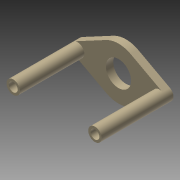
# Autodesk Inventor part: Encoder Mount
Saved by Autodesk Inventor 2013 (Build 170138000, 138)
## iProperties
Created: 2013-06-25
Part Number: Encoder Mount
Material: Generic
Document SubType Name: Modeling
Designer: mvarma
Density: 1 g/cm^3
Author: mvarma
Autodesk Inventor part; units mm, degrees
ref_plane "YZ Plane" through (0, 0, 0) normal (1, 0, 0) x (0, 1, 0)
ref_plane "XZ Plane" through (0, 0, 0) normal (0, 1, 0) x (-1, 0, 0)
ref_plane "XY Plane" through (0, 0, 0) normal (0, 0, 1) x (1, 0, 0)
sketch "Sketch1" plane through (0, 0, 0) normal (0, 0, 1) x (1, 0, 0)
  arc A0 (0, 5.3975) -> (0, -5.3975) centre (0, 0) ccw
  arc A1 (0, 11.1125) -> (0, -11.1125) centre (0, 0) ccw
  circle A2 centre (-17.4625, 0) radius 2.8702
  circle A3 centre (0, 0) radius 17.4625 construction
  line L0 (-17.4625, 0) -> (0, 0) construction
  line L1 (-18.8172, 2.5304) -> (-5.2451, 9.7968)
  line L2 (0, 0) -> (0, 11.1125)
  line L3 (0, 0) -> (0, -11.1125)
  line L4 (-18.8172, -2.5304) -> (-5.2451, -9.7968)
  dimension "d2" = 34.925
  dimension "d0" = 10.795
  dimension "d1" = 22.225
  dimension "d3" = 5.7404
  constraints: 10 end point, 8 point on circle, 4 coincident, 4 tangent, 3 centre point, 2 point on line, 1 collinear, 1 horizontal, 1 horizontal alignment, 1 perpendicular, 2 other
  measures "d0" diameter of A0
  measures "d1" diameter of A1
  measures "d3" diameter of A2
extrude "Extrusion1" add sketch "Sketch1" along normal blind 3.175 contours A0 L3 A1 L2 | A1 L4 A2 L1 | A2
extrude "Extrusion2" add sketch "Sketch1" along normal blind 30.7023 contours A2
hole "Hole1" at (-17.4625, 0, 0) direction (0, 0, 1) diameter 3.81 end through all clearance for "Flat Head Machine Screw (82)" size "#6" standard "Ansi Unified Screw Threads"
mirror "Mirror1" about plane through (0, 5.3975, 0) normal (1, 0, 0)
body "Solid1"
